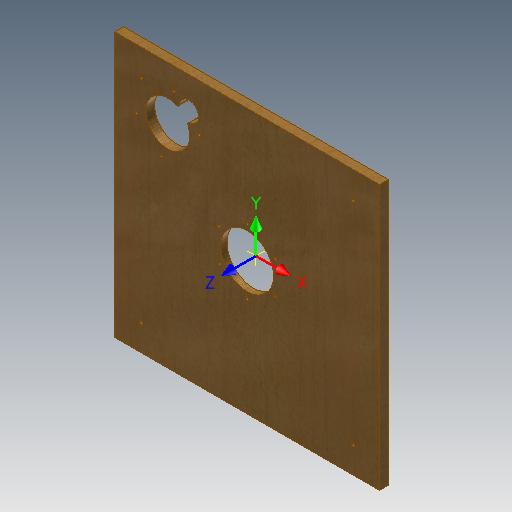
# Autodesk Inventor part: ロボットベース2019
Saved by Autodesk Inventor 2019.4 (Build 234330000, 330)
## iProperties
Created: 2018-08-09
Part Number: ロボットベース2019
Material: マツ材
Document SubType Name: Modeling
Designer: Owner
Density: 0.570257 g/cm^3
Appearance: イエロー パイン材 - 硬質 ナチュラル 抑えた光沢
Mass: 444.436 g
Surface Area: 1877.33 cm^2
Volume: 779.36 cm^3
Author: Owner
Autodesk Inventor part; units mm, degrees
ref_plane "YZ Plane" through (0, 0, 0) normal (1, 0, 0) x (0, 1, 0)
ref_plane "XZ Plane" through (0, 0, 0) normal (0, 1, 0) x (-1, 0, 0)
ref_plane "XY Plane" through (0, 0, 0) normal (0, 0, 1) x (1, 0, 0)
sketch "スケッチ1" plane through (-150, -150, 0) normal (0, 0, 1) x (1, 0, 0)
  circle A0 centre (59.9853, 240.0147) radius 24 construction
  circle A1 centre (59.9853, 240.0147) radius 24 construction
  circle A2 centre (84.0269, 264.0563) radius 10 construction
  line L0 (84.0269, 264.0563) -> (59.9853, 240.0147) construction
  line L1 (59.9853, 240.0147) -> (84.0269, 215.9731) construction
  arc A3 (84.5273, 253.0677) -> (73.0383, 264.5567) centre (84.0269, 264.0563) ccw
  arc A4 (70.2215, 262.823) -> (82.7936, 250.2509) centre (59.9853, 240.0147) ccw
  arc A5 (84.5273, 253.0677) -> (82.7936, 250.2509) centre (84.6183, 251.0698) ccw
  arc A6 (70.2215, 262.823) -> (73.0383, 264.5567) centre (71.0404, 264.6477) ccw
  line L2 (67.0564, 275.37) -> (24.63, 232.9436) construction
  line L3 (24.63, 232.9436) -> (52.9142, 204.6594) construction
  line L4 (52.9142, 204.6594) -> (95.3406, 247.0858) construction
  line L5 (95.3406, 247.0858) -> (67.0564, 275.37) construction
  line L6 (67.0564, 275.37) -> (52.9142, 204.6594) construction
  line L7 (24.63, 232.9436) -> (95.3406, 247.0858) construction
  circle A7 centre (95.3406, 247.0858) radius 1.6
  circle A8 centre (52.9142, 204.6594) radius 1.6
  circle A9 centre (24.63, 232.9436) radius 1.6
  circle A10 centre (67.0564, 275.37) radius 1.6
  line L8 (270, 30) -> (30, 30) construction
  line L9 (30, 30) -> (30, 270) construction
  line L10 (30, 270) -> (270, 270) construction
  line L11 (270, 270) -> (270, 30) construction
  line L12 (270, 30) -> (30, 270) construction
  line L13 (30, 30) -> (270, 270) construction
  circle A11 centre (30, 270) radius 2
  circle A12 centre (270, 270) radius 2
  circle A13 centre (30, 30) radius 2
  circle A14 centre (270, 30) radius 2
  circle A15 centre (150, 150) radius 30
  line L14 (150, 113) -> (117.9571, 131.5) construction
  line L15 (117.9571, 131.5) -> (117.9571, 168.5) construction
  line L16 (117.9571, 168.5) -> (150, 187) construction
  line L17 (150, 187) -> (182.0429, 168.5) construction
  line L18 (182.0429, 168.5) -> (182.0429, 131.5) construction
  line L19 (182.0429, 131.5) -> (150, 113) construction
  circle A16 centre (150, 150) radius 37 construction
  circle A17 centre (150, 113) radius 1.6
  circle A18 centre (54.1207, 93.2509) radius 1.6 construction
  line L20 (117.9571, 131.5) -> (117.9571, 168.5) construction
  line L21 (150, 113) -> (117.9571, 131.5) construction
  line L22 (117.9571, 168.5) -> (150, 187) construction
  line L23 (182.0429, 131.5) -> (150, 113) construction
  circle A19 centre (150, 150) radius 30 construction
  line L24 (150, 187) -> (182.0429, 168.5) construction
  line L25 (182.0429, 168.5) -> (182.0429, 131.5) construction
  circle A20 centre (150, 150) radius 37 construction
  circle A21 centre (182.0429, 131.5) radius 1.6
  circle A22 centre (151.2065, 38.5916) radius 1.6 construction
  line L26 (150, 113) -> (117.9571, 131.5) construction
  line L27 (182.0429, 131.5) -> (150, 113) construction
  line L28 (117.9571, 131.5) -> (117.9571, 168.5) construction
  line L29 (182.0429, 168.5) -> (182.0429, 131.5) construction
  circle A23 centre (150, 150) radius 30 construction
  line L30 (117.9571, 168.5) -> (150, 187) construction
  line L31 (150, 187) -> (182.0429, 168.5) construction
  circle A24 centre (150, 150) radius 37 construction
  circle A25 centre (182.0429, 168.5) radius 1.6
  circle A26 centre (247.0858, 95.3406) radius 1.6 construction
  line L32 (182.0429, 131.5) -> (150, 113) construction
  line L33 (182.0429, 168.5) -> (182.0429, 131.5) construction
  line L34 (150, 113) -> (117.9571, 131.5) construction
  line L35 (150, 187) -> (182.0429, 168.5) construction
  circle A27 centre (150, 150) radius 30 construction
  line L36 (117.9571, 131.5) -> (117.9571, 168.5) construction
  line L37 (117.9571, 168.5) -> (150, 187) construction
  circle A28 centre (150, 150) radius 37 construction
  circle A29 centre (150, 187) radius 1.6
  circle A30 centre (245.8793, 206.7491) radius 1.6 construction
  line L38 (182.0429, 168.5) -> (182.0429, 131.5) construction
  line L39 (150, 187) -> (182.0429, 168.5) construction
  line L40 (182.0429, 131.5) -> (150, 113) construction
  line L41 (117.9571, 168.5) -> (150, 187) construction
  circle A31 centre (150, 150) radius 30 construction
  line L42 (150, 113) -> (117.9571, 131.5) construction
  line L43 (117.9571, 131.5) -> (117.9571, 168.5) construction
  circle A32 centre (150, 150) radius 37 construction
  circle A33 centre (117.9571, 168.5) radius 1.6
  circle A34 centre (148.7935, 261.4084) radius 1.6 construction
  line L44 (150, 187) -> (182.0429, 168.5) construction
  line L45 (117.9571, 168.5) -> (150, 187) construction
  line L46 (182.0429, 168.5) -> (182.0429, 131.5) construction
  line L47 (117.9571, 131.5) -> (117.9571, 168.5) construction
  circle A35 centre (150, 150) radius 30 construction
  line L48 (182.0429, 131.5) -> (150, 113) construction
  line L49 (150, 113) -> (117.9571, 131.5) construction
  circle A36 centre (150, 150) radius 37 construction
  circle A37 centre (117.9571, 131.5) radius 1.6
  line L50 (0, 300) -> (300, 300)
  line L51 (300, 300) -> (300, 0)
  line L52 (300, 0) -> (0, 0)
  line L53 (0, 0) -> (0, 300)
  line L54 (0, 300) -> (300, 0) construction
  line L55 (300, 300) -> (0, 0) construction
  point P0 (150, 150)
  point P1 (81.1985, 261.2279)
  point P2 (150, 150)
  point P3 (59.8791, 125.8522)
  point P4 (150, 150)
  point P5 (125.8522, 59.8791)
  point P6 (150, 150)
  point P7 (215.9731, 84.0269)
  point P8 (150, 150)
  point P9 (240.1209, 174.1478)
  point P10 (150, 150)
  point P11 (174.1478, 240.1209)
  dimension "d30" = 74
  dimension "d6" = 48
  dimension "d7" = 20
  dimension "d10" = 25
  dimension "d11" = 11
  dimension "d12" = 2
  dimension "d15" = 40
  dimension "d16" = 60
  dimension "d17" = 3.2
  dimension "d18" = 240
  dimension "d19" = 4
  dimension "d22" = 240
  dimension "d25" = 240
  dimension "d28" = 60
  dimension "d31" = 3.2
  dimension "d34" = 360
  dimension "d36" = 300
  dimension "d39" = 127.3
  dimension "d40" = 3.2
  dimension "d41" = 48
  constraints: 112 end point, 39 coincident, 32 centre point, 8 midpoint, 8 point on circle, 7 perpendicular, 6 parallel, 5 tangent, 3 equal radius, 3 horizontal, 3 point on line, 3 vertical alignment, 1 vertical, 185 other
  measures "d6" diameter of A1
  measures "d7" diameter of A2
  measures "d10" radius of A4
  measures "d11" radius of A3
  measures "d12" radius of A5
  measures "d15" distance of L2.end L3.end
  measures "d16" distance of L2.start L2.end
  measures "d17" diameter of A7
  measures "d18" distance of L8.end L9.end
  measures "d19" diameter of A11
  measures "d22" distance of A11.centre A12.centre
  measures "d25" distance of A11.centre A13.centre
  measures "d28" diameter of A15
  measures "d31" diameter of A17
  measures "d36" distance of L51.end L52.end
  measures "d39" distance of point (150, 150) A0.centre
  measures "d40" diameter of A10
  measures "d41" diameter of A0
extrude "押し出し2" add sketch "スケッチ1" along normal blind 10
sketch "スケッチ2" plane through (-150, -150, 0) normal (0, 0, -1) x (-1, 0, 0)
  circle A0 centre (-150, 150) radius 90
  dimension "d42" = 180
  constraints: 1 centre point, 1 coincident
  measures "d42" diameter of A0
extrude "押し出し3" cut sketch "スケッチ2" against normal blind 3
